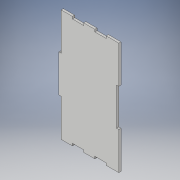
# Autodesk Inventor part: Pared Garita
Saved by Autodesk Inventor 2019 (Build 230136000, 136)
## iProperties
Created: 2020-03-09
Part Number: Pared Garita
Material: Genérico
Document SubType Name: Modeling
Designer: Diego Guillén
Density: 1 g/cm^3
Appearance: Valor por defecto
Author: Diego Guillén
Autodesk Inventor part; units mm, degrees
ref_plane "YZ Plane" through (0, 0, 0) normal (1, 0, 0) x (0, 1, 0)
ref_plane "XZ Plane" through (0, 0, 0) normal (0, 1, 0) x (-1, 0, 0)
ref_plane "XY Plane" through (0, 0, 0) normal (0, 0, 1) x (1, 0, 0)
sketch "Boceto1" plane through (0, 0, 0) normal (0, 0, 1) x (1, 0, 0)
  line L0 (0, 0) -> (80, 0)
  line L1 (80, 0) -> (80, 150)
  line L2 (80, 150) -> (0, 150)
  line L3 (0, 150) -> (0, 0)
  dimension "d0" = 80
  dimension "d1" = 150
  constraints: 8 end point, 2 parallel, 1 horizontal, 1 perpendicular
  measures "d0" distance of L1.end L2.end
  measures "d1" distance of L0.end L1.end
extrude "Extrusión1" add sketch "Boceto1" along normal blind 3
sketch "Boceto2" plane through (0, 0, 3) normal (0, 0, 1) x (1, 0, 0)
  line L0 (0, 0) -> (80, 0) construction
  line L1 (80, 0) -> (80, 150) construction
  line L2 (80, 150) -> (0, 150) construction
  line L3 (0, 150) -> (0, 0) construction
  line L4 (3, 0) -> (0, 0)
  line L5 (0, 0) -> (0, 50)
  line L6 (0, 50) -> (3, 50)
  line L7 (3, 50) -> (3, 0)
  line L8 (0, 150) -> (3, 150)
  line L9 (3, 150) -> (3, 100)
  line L10 (3, 100) -> (0, 100)
  line L11 (0, 100) -> (0, 150)
  line L12 (77, 100) -> (80, 100)
  line L13 (80, 100) -> (80, 50)
  line L14 (80, 50) -> (77, 50)
  line L15 (77, 50) -> (77, 100)
  line L16 (80, 0) -> (80, 150) construction
  point P0 (80, 75)
  point P1 (80, 75)
  dimension "d4" = 3
  dimension "d5" = 50
  dimension "d6" = 3
  dimension "d7" = 50
  dimension "d8" = 50
  dimension "d9" = 3
  constraints: 24 end point, 6 parallel, 3 horizontal, 3 perpendicular, 2 coincident, 2 midpoint, 1 collinear
  measures "d4" distance of L5.end L6.end
  measures "d5" distance of L6.end L4.start
  measures "d6" distance of L9.end L10.end
  measures "d7" distance of L8.end L9.end
  measures "d8" distance of L14.end L12.start
  measures "d9" distance of L13.end L14.end
extrude "Extrusión2" cut sketch "Boceto2" against normal blind 3
sketch "Boceto3" plane through (0, 0, 3) normal (0, 0, 1) x (1, 0, 0)
  line L0 (3, 50) -> (3, 0) construction
  line L1 (3, 0) -> (80, 0) construction
  line L2 (80, 0) -> (80, 50) construction
  line L3 (80, 50) -> (77, 50) construction
  line L4 (77, 50) -> (77, 100) construction
  line L5 (77, 100) -> (80, 100) construction
  line L6 (80, 100) -> (80, 150) construction
  line L7 (80, 150) -> (3, 150) construction
  line L8 (3, 150) -> (3, 100) construction
  line L9 (3, 100) -> (0, 100) construction
  line L10 (0, 100) -> (0, 50) construction
  line L11 (0, 50) -> (3, 50) construction
  line L12 (18, 3) -> (33, 3)
  line L13 (33, 3) -> (33, 0)
  line L14 (33, 0) -> (18, 0)
  line L15 (18, 0) -> (18, 3)
  line L16 (48, 3) -> (63, 3)
  line L17 (63, 3) -> (63, 0)
  line L18 (63, 0) -> (48, 0)
  line L19 (48, 0) -> (48, 3)
  line L20 (3, 0) -> (80, 0) construction
  line L21 (18, 150) -> (33, 150)
  line L22 (33, 150) -> (33, 147)
  line L23 (33, 147) -> (18, 147)
  line L24 (18, 147) -> (18, 150)
  line L25 (48, 147) -> (63, 147)
  line L26 (63, 147) -> (63, 150)
  line L27 (63, 150) -> (48, 150)
  line L28 (48, 150) -> (48, 147)
  line L29 (80, 150) -> (3, 150) construction
  point P0 (0, 0)
  dimension "d12" = 3
  dimension "d13" = 15
  dimension "d14" = 15
  dimension "d15" = 3
  dimension "d16" = 15
  dimension "d17" = 15
  dimension "d20" = 3
  dimension "d21" = 3
  dimension "d22" = 15
  dimension "d23" = 15
  dimension "d24" = 15
  dimension "d25" = 15
  constraints: 32 end point, 8 parallel, 4 horizontal, 4 perpendicular, 3 collinear, 2 point on line
  measures "d12" distance of L12.end L13.end
  measures "d13" distance of L12.start L12.end
  measures "d14" distance of L16.start L16.end
  measures "d15" distance of L16.end L17.end
  measures "d16" distance between parallel lines of L19 L13
  measures "d17" distance between parallel lines of L0 L15
  measures "d20" distance of L21.end L22.end
  measures "d21" distance of L25.end L26.end
  measures "d22" distance of L27.end L21.end
  measures "d23" distance from line of L8 L21.start
  measures "d24" distance of L25.start L25.end
  measures "d25" distance of L22.end L23.end
extrude "Extrusión3" cut sketch "Boceto3" against normal blind 10 contours L12 L13 L14 L15 | L16 L17 L18 L19
sketch "Boceto4" plane through (0, 0, 3) normal (0, 0, 1) x (1, 0, 0)
  line L0 (33, 3) -> (33, 0) construction
  line L1 (33, 0) -> (48, 0) construction
  line L2 (48, 0) -> (48, 3) construction
  line L3 (48, 3) -> (63, 3) construction
  line L4 (63, 3) -> (63, 0) construction
  line L5 (63, 0) -> (80, 0) construction
  line L6 (80, 0) -> (80, 50) construction
  line L7 (80, 50) -> (77, 50) construction
  line L8 (77, 50) -> (77, 100) construction
  line L9 (77, 100) -> (80, 100) construction
  line L10 (80, 100) -> (80, 150) construction
  line L11 (80, 150) -> (3, 150) construction
  line L12 (3, 150) -> (3, 100) construction
  line L13 (3, 100) -> (0, 100) construction
  line L14 (0, 100) -> (0, 50) construction
  line L15 (0, 50) -> (3, 50) construction
  line L16 (3, 50) -> (3, 0) construction
  line L17 (3, 0) -> (18, 0) construction
  line L18 (18, 0) -> (18, 3) construction
  line L19 (18, 3) -> (33, 3) construction
  line L20 (18, 150) -> (33, 150)
  line L21 (33, 150) -> (33, 147)
  line L22 (33, 147) -> (18, 147)
  line L23 (18, 147) -> (18, 150)
  line L24 (48, 150) -> (63, 150)
  line L25 (63, 150) -> (63, 147)
  line L26 (63, 147) -> (48, 147)
  line L27 (48, 147) -> (48, 150)
  line L28 (80, 150) -> (3, 150) construction
  point P0 (0, 0)
  dimension "d26" = 15
  dimension "d27" = 15
  dimension "d28" = 15
  dimension "d29" = 15
  dimension "d30" = 3
  constraints: 16 end point, 4 parallel, 2 horizontal, 2 perpendicular, 2 point on line, 1 collinear
  measures "d26" distance between parallel lines of L12 L23
  measures "d27" distance of L21.end L22.end
  measures "d28" distance between parallel lines of L27 L21
  measures "d29" distance of L25.end L26.end
  measures "d30" distance of L22.end L20.start
extrude "Extrusión4" cut sketch "Boceto4" against normal blind 10
equation "\"d6\" = d4"
equation "\"d7\" = d5"
equation "\"d8\" = d7"
equation "\"d9\" = d4"
